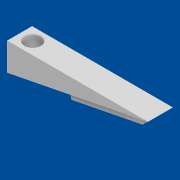
# Autodesk Inventor part: GRIPPER2
Saved by Autodesk Inventor 2020 (Build 240168000, 168)
## iProperties
Created: 2022-02-12
Part Number: GRIPPER2
Material: Generic
Document SubType Name: Modeling
Designer: niladri
Density: 1 g/cm^3
Appearance: Default
Author: niladri
Autodesk Inventor part; units mm, degrees
ref_plane "YZ Plane" through (0, 0, 0) normal (1, 0, 0) x (0, 1, 0)
ref_plane "XZ Plane" through (0, 0, 0) normal (0, 1, 0) x (-1, 0, 0)
ref_plane "XY Plane" through (0, 0, 0) normal (0, 0, 1) x (1, 0, 0)
sketch "Sketch1" plane through (0, 0, 0) normal (0, 0, 1) x (1, 0, 0)
  line L0 (-15.9265, 7.9959) -> (-1.5469, 7.9959)
  line L1 (-15.9265, 5.1636) -> (-15.9265, 7.9959)
  line L2 (-15.9265, 5.1636) -> (-1.5469, 7.9959)
  point P0 (0, 0)
  constraints: 6 end point, 1 horizontal
extrude "Extrusion1" add sketch "Sketch1" along normal blind 2.54
sketch "Sketch2" plane through (-1.5469, 7.9959, 0) normal (0.1932565, -0.9811483, 0) x (0.9811483, 0.1932565, 0)
  line L0 (-1.1823, 2.0698) -> (-8.5899, 2.0698)
  line L1 (-8.5899, 2.0698) -> (-8.5899, 0.4575)
  line L2 (-8.5899, 0.4575) -> (-1.1823, 0.4575)
  line L3 (-1.1823, 0.4575) -> (-1.1823, 2.0698)
  point P0 (-0.0275, 0)
  constraints: 8 end point, 2 parallel, 1 horizontal, 1 perpendicular
extrude "Extrusion2" add sketch "Sketch2" along normal blind 0.762
sketch "Sketch3" plane through (-15.9265, 7.9959, 0) normal (0, 1, 0) x (1, 0, 0)
  circle A0 centre (1.3508, -1.2855) radius 0.8416
  point P0 (15.9265, 0)
  constraints: 1 centre point
extrude "Extrusion3" cut sketch "Sketch3" against normal blind 12.7
body "Solid1"
